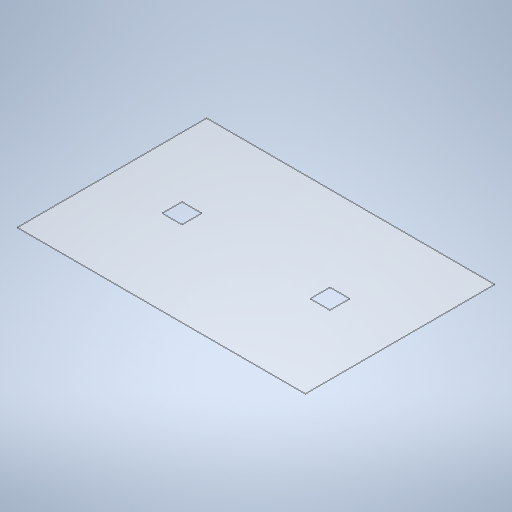
# Autodesk Inventor part: Base
Saved by Autodesk Inventor 2025.1 (Build 291241000, 241)
## iProperties
Created: 2024-09-06
Part Number: Base
Material: Acrylic
Document SubType Name: Modeling
Designer: joser
Density: 1.188 g/cm^3
Appearance: Transparent - Clear
Author: joser
Autodesk Inventor part; units mm, degrees
ref_plane "YZ Plane" through (0, 0, 0) normal (1, 0, 0) x (0, 1, 0)
ref_plane "XZ Plane" through (0, 0, 0) normal (0, 1, 0) x (-1, 0, 0)
ref_plane "XY Plane" through (0, 0, 0) normal (0, 0, 1) x (1, 0, 0)
sketch "Sketch1" plane through (0, 0, 0) normal (0, 1, 0) x (-1, 0, 0)
  line L0 (-584, 384) -> (584, 384)
  line L1 (584, 384) -> (584, -384)
  line L2 (584, -384) -> (-584, -384)
  line L3 (-584, -384) -> (-584, 384)
  line L4 (-584, 384) -> (584, -384) construction
  line L5 (584, 384) -> (-584, -384) construction
  line L6 (340, 40) -> (260, 40)
  line L7 (260, 40) -> (260, -40)
  line L8 (260, -40) -> (340, -40)
  line L9 (340, -40) -> (340, 40)
  line L10 (340, 40) -> (260, -40) construction
  line L11 (260, 40) -> (340, -40) construction
  line L12 (-340, -40) -> (-260, -40)
  line L13 (-340, 40) -> (-340, -40)
  line L14 (-260, 40) -> (-340, 40)
  line L15 (-260, -40) -> (-260, 40)
  point P0 (0, 0)
  point P1 (300, 0)
  dimension "d0" = 1168
  dimension "d1" = 768
  dimension "d13" = 300
  dimension "d14" = 80
  dimension "d15" = 80
  dimension "d18" = 600
  constraints: 32 end point, 4 midpoint, 4 parallel, 3 horizontal, 2 perpendicular, 1 horizontal alignment, 8 other
  measures "d0" distance of L1.end L2.end
  measures "d1" distance of L0.end L1.end
  measures "d13" distance of point (0, 0) point (300, 0)
  measures "d14" distance of L7.end L8.end
  measures "d15" distance of L6.end L7.end
  measures "d18" distance of L7.end L12.start
extrude "Extrusion1" add sketch "Sketch1" along normal mid plane 3
equation "\"d15\" = d14"
body "Solid1"
